Autodesk Fusion 360 part; units mm, degrees
(part 8 of 9)
  spline S40 degree 5 poles (-3.0485, 6.2691) (-3.0485, 6.2692) (-3.0485, 6.2692) (-3.0486, 6.2693) (-3.0487, 6.2695) (-3.0488, 6.2697) (-3.0489, 6.27) (-3.0491, 6.2703) (-3.0493, 6.2707) (-3.0495, 6.271) (-3.0497, 6.2715) (-3.0499, 6.2719) (-3.0502, 6.2724) (-3.0504, 6.2729) (-3.0507, 6.2734) (-3.051, 6.274) (-3.0514, 6.2746) (-3.0517, 6.2752) (-3.0521, 6.2759) (-3.0525, 6.2766) (-3.0529, 6.2773) (-3.0533, 6.2781) (-3.0537, 6.2789) (-3.0542, 6.2797) (-3.0547, 6.2806) (-3.0552, 6.2815) (-3.0557, 6.2824) (-3.0562, 6.2833) (-3.0568, 6.2843) (-3.0574, 6.2853) (-3.058, 6.2863) (-3.0586, 6.2874) (-3.0592, 6.2885) (-3.0599, 6.2896) (-3.0606, 6.2907) (-3.0613, 6.2919) (-3.062, 6.2931) (-3.0627, 6.2943) (-3.0635, 6.2955) (-3.0643, 6.2968) (-3.0651, 6.2981) (-3.0659, 6.2994) (-3.0667, 6.3008) (-3.0676, 6.3022) (-3.0684, 6.3036) (-3.0693, 6.305) (-3.0703, 6.3065) (-3.0712, 6.308) (-3.0722, 6.3095) (-3.0731, 6.311) (-3.0742, 6.3125) (-3.0752, 6.3141) (-3.0762, 6.3157) (-3.0773, 6.3174) (-3.0784, 6.319) (-3.0795, 6.3207) (-3.0806, 6.3224) (-3.0817, 6.3241) (-3.0829, 6.3259) (-3.0841, 6.3276) (-3.0853, 6.3294) (-3.0865, 6.3312) (-3.0878, 6.3331) (-3.0891, 6.3349) (-3.0904, 6.3368) (-3.0917, 6.3387) (-3.093, 6.3406) (-3.0944, 6.3426) (-3.0957, 6.3445) (-3.0971, 6.3465) (-3.0986, 6.3485) (-3.1, 6.3505) (-3.1015, 6.3526) (-3.1029, 6.3546) (-3.1044, 6.3567) (-3.106, 6.3588) (-3.1075, 6.361) (-3.1091, 6.3631) (-3.1107, 6.3653) (-3.1123, 6.3675) (-3.1139, 6.3697) (-3.1156, 6.3719) (-3.1173, 6.3741) (-3.119, 6.3764) (-3.1207, 6.3787) (-3.1224, 6.381) (-3.1242, 6.3833) (-3.126, 6.3856) (-3.1278, 6.388) (-3.1296, 6.3904) (-3.1314, 6.3927) (-3.1333, 6.3951) (-3.1352, 6.3976) (-3.1371, 6.4) (-3.139, 6.4025) (-3.141, 6.4049) (-3.143, 6.4074) (-3.145, 6.4099) (-3.147, 6.4125) (-3.149, 6.415) (-3.1511, 6.4176) (-3.1532, 6.4201) (-3.1553, 6.4227) (-3.1574, 6.4253) (-3.1596, 6.4279) (-3.1617, 6.4306) (-3.1639, 6.4332) (-3.1662, 6.4359) (-3.1684, 6.4386) (-3.1707, 6.4413) (-3.1729, 6.444) (-3.1752, 6.4467) (-3.1776, 6.4494) (-3.1799, 6.4522) (-3.1823, 6.4549) (-3.1847, 6.4577) (-3.1871, 6.4605) (-3.1895, 6.4633) (-3.192, 6.4661) (-3.1945, 6.469) (-3.197, 6.4718) (-3.1995, 6.4747) (-3.202, 6.4776) (-3.2046, 6.4805) (-3.2072, 6.4834) (-3.2098, 6.4863) (-3.2124, 6.4892) (-3.2151, 6.4921) (-3.2178, 6.4951) (-3.2205, 6.498) (-3.2232, 6.501) (-3.2259, 6.504) (-3.2287, 6.507) (-3.2315, 6.51) (-3.2343, 6.513) (-3.2371, 6.5161) (-3.24, 6.5191) (-3.2428, 6.5222) (-3.2457, 6.5252) (-3.2487, 6.5283) (-3.2516, 6.5314) (-3.2546, 6.5345) (-3.2576, 6.5376) (-3.2606, 6.5408) (-3.2636, 6.5439) (-3.2666, 6.547) (-3.2697, 6.5502) (-3.2728, 6.5533) (-3.2759, 6.5565) (-3.2791, 6.5597) (-3.2822, 6.5629) (-3.2854, 6.5661) (-3.2886, 6.5693) (-3.2918, 6.5725) (-3.2951, 6.5758) (-3.2984, 6.579) (-3.3017, 6.5822) (-3.305, 6.5855) (-3.3083, 6.5888) (-3.3117, 6.592) (-3.3151, 6.5953) (-3.3185, 6.5986) (-3.3219, 6.6019) (-3.3253, 6.6052) (-3.3288, 6.6085) (-3.3323, 6.6119) (-3.3358, 6.6152) (-3.3393, 6.6186) (-3.3429, 6.6219) (-3.3465, 6.6253) (-3.3501, 6.6286) (-3.3537, 6.632) (-3.3573, 6.6354) (-3.361, 6.6388) (-3.3647, 6.6422) (-3.3684, 6.6456) (-3.3721, 6.649) (-3.3759, 6.6524) (-3.3797, 6.6558) (-3.3835, 6.6592) (-3.3873, 6.6627) (-3.3911, 6.6661) (-3.395, 6.6695) (-3.3989, 6.673) (-3.4028, 6.6765) (-3.4067, 6.6799) (-3.4107, 6.6834) (-3.4147, 6.6869) (-3.4187, 6.6904) (-3.4227, 6.6939) (-3.4267, 6.6973) (-3.4308, 6.7008) (-3.4349, 6.7044) (-3.439, 6.7079) (-3.4431, 6.7114) (-3.4472, 6.7149) (-3.4514, 6.7184) (-3.4556, 6.722) (-3.4598, 6.7255) (-3.464, 6.729) (-3.4683, 6.7326) (-3.4726, 6.7361) (-3.4769, 6.7397) (-3.4812, 6.7432) (-3.4856, 6.7468) (-3.4899, 6.7504) (-3.4943, 6.7539) (-3.4987, 6.7575) (-3.5031, 6.7611) (-3.5076, 6.7647) (-3.5121, 6.7683) (-3.5166, 6.7719) (-3.5211, 6.7754) (-3.5256, 6.779) (-3.5302, 6.7826) (-3.5348, 6.7862) (-3.5394, 6.7899) (-3.544, 6.7935) (-3.5486, 6.7971) (-3.5533, 6.8007) (-3.558, 6.8043) (-3.5627, 6.8079) (-3.5674, 6.8116) (-3.5722, 6.8152) (-3.577, 6.8188) (-3.5818, 6.8224) (-3.5866, 6.8261) (-3.5914, 6.8297) (-3.5963, 6.8334) (-3.6012, 6.837) (-3.6061, 6.8406) (-3.611, 6.8443) (-3.616, 6.8479) (-3.6209, 6.8516) (-3.6259, 6.8552) (-3.6309, 6.8589) (-3.636, 6.8625) (-3.641, 6.8662) (-3.6461, 6.8698) (-3.6512, 6.8735) (-3.6563, 6.8772) (-3.6604, 6.8801) (-3.6635, 6.8823) (-3.6656, 6.8837) (-3.6666, 6.8845) knots 0 0 0 0 0 0 0.00416667 0.00833333 0.0125 0.01666667 0.02083333 0.025 0.02916667 0.03333333 0.0375 0.04166667 0.04583333 0.05 0.05416667 0.05833333 0.0625 0.06666667 0.07083333 0.075 0.07916667 0.08333333 0.0875 0.09166667 0.09583333 0.1 0.10416667 0.10833333 0.1125 0.11666667 0.12083333 0.125 0.12916667 0.13333333 0.1375 0.14166667 0.14583333 0.15 0.15416667 0.15833333 0.1625 0.16666667 0.17083333 0.175 0.17916667 0.18333333 0.1875 0.19166667 0.19583333 0.2 0.20416667 0.20833333 0.2125 0.21666667 0.22083333 0.225 0.22916667 0.23333333 0.2375 0.24166667 0.24583333 0.25 0.25416667 0.25833333 0.2625 0.26666667 0.27083333 0.275 0.27916667 0.28333333 0.2875 0.29166667 0.29583333 0.3 0.30416667 0.30833333 0.3125 0.31666667 0.32083333 0.325 0.32916667 0.33333333 0.3375 0.34166667 0.34583333 0.35 0.35416667 0.35833333 0.3625 0.36666667 0.37083333 0.375 0.37916667 0.38333333 0.3875 0.39166667 0.39583333 0.4 0.40416667 0.40833333 0.4125 0.41666667 0.42083333 0.425 0.42916667 0.43333333 0.4375 0.44166667 0.44583333 0.45 0.45416667 0.45833333 0.4625 0.46666667 0.47083333 0.475 0.47916667 0.48333333 0.4875 0.49166667 0.49583333 0.5 0.50416667 0.50833333 0.5125 0.51666667 0.52083333 0.525 0.52916667 0.53333333 0.5375 0.54166667 0.54583333 0.55 0.55416667 0.55833333 0.5625 0.56666667 0.57083333 0.575 0.57916667 0.58333333 0.5875 0.59166667 0.59583333 0.6 0.60416667 0.60833333 0.6125 0.61666667 0.62083333 0.625 0.62916667 0.63333333 0.6375 0.64166667 0.64583333 0.65 0.65416667 0.65833333 0.6625 0.66666667 0.67083333 0.675 0.67916667 0.68333333 0.6875 0.69166667 0.69583333 0.7 0.70416667 0.70833333 0.7125 0.71666667 0.72083333 0.725 0.72916667 0.73333333 0.7375 0.74166667 0.74583333 0.75 0.75416667 0.75833333 0.7625 0.76666667 0.77083333 0.775 0.77916667 0.78333333 0.7875 0.79166667 0.79583333 0.8 0.80416667 0.80833333 0.8125 0.81666667 0.82083333 0.825 0.82916667 0.83333333 0.8375 0.84166667 0.84583333 0.85 0.85416667 0.85833333 0.8625 0.86666667 0.87083333 0.875 0.87916667 0.88333333 0.8875 0.89166667 0.89583333 0.9 0.90416667 0.90833333 0.9125 0.91666667 0.92083333 0.925 0.92916667 0.93333333 0.9375 0.94166667 0.94583333 0.95 0.95416667 0.95833333 0.9625 0.96666667 0.97083333 0.975 0.97916667 0.98333333 0.9875 0.99166667 0.99583333 1 1 1 1 1 1
  arc A41 (-3.6666, 6.8845) -> (-4.1288, 6.6176) centre (0, 0) ccw
  spline S41 degree 5 poles (-4.1288, 6.6176) (-4.1287, 6.6163) (-4.1285, 6.6138) (-4.1281, 6.61) (-4.1276, 6.605) (-4.127, 6.5988) (-4.1264, 6.5925) (-4.1258, 6.5863) (-4.1251, 6.5801) (-4.1245, 6.5739) (-4.1238, 6.5677) (-4.1232, 6.5616) (-4.1225, 6.5555) (-4.1218, 6.5494) (-4.1211, 6.5433) (-4.1204, 6.5372) (-4.1197, 6.5312) (-4.119, 6.5251) (-4.1183, 6.5191) (-4.1175, 6.5131) (-4.1168, 6.5072) (-4.116, 6.5012) (-4.1153, 6.4953) (-4.1145, 6.4894) (-4.1137, 6.4835) (-4.1129, 6.4776) (-4.1121, 6.4718) (-4.1113, 6.4659) (-4.1105, 6.4601) (-4.1097, 6.4543) (-4.1089, 6.4486) (-4.108, 6.4428) (-4.1072, 6.4371) (-4.1063, 6.4314) (-4.1055, 6.4257) (-4.1046, 6.42) (-4.1037, 6.4144) (-4.1028, 6.4087) (-4.1019, 6.4031) (-4.101, 6.3975) (-4.1001, 6.392) (-4.0992, 6.3864) (-4.0983, 6.3809) (-4.0974, 6.3754) (-4.0964, 6.3699) (-4.0955, 6.3645) (-4.0945, 6.359) (-4.0936, 6.3536) (-4.0926, 6.3482) (-4.0917, 6.3428) (-4.0907, 6.3375) (-4.0897, 6.3322) (-4.0887, 6.3268) (-4.0877, 6.3216) (-4.0867, 6.3163) (-4.0857, 6.311) (-4.0847, 6.3058) (-4.0837, 6.3006) (-4.0827, 6.2954) (-4.0816, 6.2903) (-4.0806, 6.2851) (-4.0795, 6.28) (-4.0785, 6.2749) (-4.0774, 6.2699) (-4.0764, 6.2648) (-4.0753, 6.2598) (-4.0743, 6.2548) (-4.0732, 6.2498) (-4.0721, 6.2448) (-4.071, 6.2399) (-4.0699, 6.235) (-4.0688, 6.2301) (-4.0677, 6.2252) (-4.0666, 6.2204) (-4.0655, 6.2156) (-4.0644, 6.2108) (-4.0633, 6.206) (-4.0622, 6.2012) (-4.061, 6.1965) (-4.0599, 6.1918) (-4.0588, 6.1871) (-4.0576, 6.1824) (-4.0565, 6.1778) (-4.0553, 6.1732) (-4.0542, 6.1686) (-4.053, 6.164) (-4.0519, 6.1595) (-4.0507, 6.1549) (-4.0496, 6.1504) (-4.0484, 6.146) (-4.0472, 6.1415) (-4.0461, 6.1371) (-4.0449, 6.1327) (-4.0437, 6.1283) (-4.0425, 6.1239) (-4.0413, 6.1196) (-4.0401, 6.1153) (-4.039, 6.111) (-4.0378, 6.1067) (-4.0366, 6.1025) (-4.0354, 6.0983) (-4.0342, 6.0941) (-4.033, 6.0899) (-4.0318, 6.0858) (-4.0306, 6.0817) (-4.0294, 6.0776) (-4.0282, 6.0735) (-4.0269, 6.0695) (-4.0257, 6.0655) (-4.0245, 6.0615) (-4.0233, 6.0575) (-4.0221, 6.0536) (-4.0209, 6.0496) (-4.0197, 6.0457) (-4.0185, 6.0419) (-4.0172, 6.038) (-4.016, 6.0342) (-4.0148, 6.0304) (-4.0136, 6.0266) (-4.0124, 6.0229) (-4.0112, 6.0192) (-4.0099, 6.0155) (-4.0087, 6.0118) (-4.0075, 6.0082) (-4.0063, 6.0046) (-4.0051, 6.001) (-4.0039, 5.9974) (-4.0026, 5.9939) (-4.0014, 5.9904) (-4.0002, 5.9869) (-3.999, 5.9834) (-3.9978, 5.98) (-3.9966, 5.9766) (-3.9954, 5.9732) (-3.9942, 5.9698) (-3.993, 5.9665) (-3.9918, 5.9632) (-3.9906, 5.9599) (-3.9894, 5.9567) (-3.9882, 5.9534) (-3.987, 5.9502) (-3.9858, 5.9471) (-3.9846, 5.9439) (-3.9834, 5.9408) (-3.9822, 5.9377) (-3.981, 5.9346) (-3.9799, 5.9316) (-3.9787, 5.9286) (-3.9775, 5.9256) (-3.9763, 5.9226) (-3.9752, 5.9197) (-3.974, 5.9168) (-3.9729, 5.9139) (-3.9717, 5.9111) (-3.9706, 5.9083) (-3.9694, 5.9055) (-3.9683, 5.9027) (-3.9671, 5.9) (-3.966, 5.8973) (-3.9649, 5.8946) (-3.9638, 5.8919) (-3.9626, 5.8893) (-3.9615, 5.8867) (-3.9604, 5.8841) (-3.9593, 5.8816) (-3.9582, 5.8791) (-3.9572, 5.8766) (-3.9561, 5.8741) (-3.955, 5.8717) (-3.9539, 5.8693) (-3.9529, 5.8669) (-3.9518, 5.8646) (-3.9508, 5.8622) (-3.9497, 5.8599) (-3.9487, 5.8577) (-3.9477, 5.8555) (-3.9466, 5.8532) (-3.9456, 5.8511) (-3.9446, 5.8489) (-3.9436, 5.8468) (-3.9426, 5.8447) (-3.9417, 5.8427) (-3.9407, 5.8406) (-3.9397, 5.8386) (-3.9388, 5.8367) (-3.9378, 5.8347) (-3.9369, 5.8328) (-3.936, 5.8309) (-3.935, 5.8291) (-3.9341, 5.8272) (-3.9332, 5.8254) (-3.9324, 5.8237) (-3.9315, 5.8219) (-3.9306, 5.8202) (-3.9298, 5.8186) (-3.9289, 5.8169) (-3.9281, 5.8153) (-3.9272, 5.8137) (-3.9264, 5.8122) (-3.9256, 5.8106) (-3.9248, 5.8091) (-3.9241, 5.8077) (-3.9233, 5.8062) (-3.9225, 5.8048) (-3.9218, 5.8035) (-3.9211, 5.8021) (-3.9204, 5.8008) (-3.9197, 5.7995) (-3.919, 5.7983) (-3.9183, 5.7971) (-3.9176, 5.7959) (-3.917, 5.7947) (-3.9163, 5.7936) (-3.9157, 5.7925) (-3.9151, 5.7914) (-3.9145, 5.7904) (-3.914, 5.7894) (-3.9134, 5.7884) (-3.9128, 5.7875) (-3.9123, 5.7866) (-3.9118, 5.7857) (-3.9113, 5.7849) (-3.9108, 5.7841) (-3.9104, 5.7833) (-3.9099, 5.7825) (-3.9095, 5.7818) (-3.9091, 5.7811) (-3.9087, 5.7805) (-3.9083, 5.7799) (-3.9079, 5.7793) (-3.9076, 5.7787) (-3.9073, 5.7782) (-3.9069, 5.7777) (-3.9067, 5.7773) (-3.9064, 5.7768) (-3.9061, 5.7764) (-3.9059, 5.7761) (-3.9057, 5.7758) (-3.9055, 5.7755) (-3.9053, 5.7752) (-3.9052, 5.775) (-3.9051, 5.7748) (-3.905, 5.7747) (-3.905, 5.7747) (-3.905, 5.7746) knots -1 -1 -1 -1 -1 -1 -0.99583333 -0.99166667 -0.9875 -0.98333333 -0.97916667 -0.975 -0.97083333 -0.96666667 -0.9625 -0.95833333 -0.95416667 -0.95 -0.94583333 -0.94166667 -0.9375 -0.93333333 -0.92916667 -0.925 -0.92083333 -0.91666667 -0.9125 -0.90833333 -0.90416667 -0.9 -0.89583333 -0.89166667 -0.8875 -0.88333333 -0.87916667 -0.875 -0.87083333 -0.86666667 -0.8625 -0.85833333 -0.85416667 -0.85 -0.84583333 -0.84166667 -0.8375 -0.83333333 -0.82916667 -0.825 -0.82083333 -0.81666667 -0.8125 -0.80833333 -0.80416667 -0.8 -0.79583333 -0.79166667 -0.7875 -0.78333333 -0.77916667 -0.775 -0.77083333 -0.76666667 -0.7625 -0.75833333 -0.75416667 -0.75 -0.74583333 -0.74166667 -0.7375 -0.73333333 -0.72916667 -0.725 -0.72083333 -0.71666667 -0.7125 -0.70833333 -0.70416667 -0.7 -0.69583333 -0.69166667 -0.6875 -0.68333333 -0.67916667 -0.675 -0.67083333 -0.66666667 -0.6625 -0.65833333 -0.65416667 -0.65 -0.64583333 -0.64166667 -0.6375 -0.63333333 -0.62916667 -0.625 -0.62083333 -0.61666667 -0.6125 -0.60833333 -0.60416667 -0.6 -0.59583333 -0.59166667 -0.5875 -0.58333333 -0.57916667 -0.575 -0.57083333 -0.56666667 -0.5625 -0.55833333 -0.55416667 -0.55 -0.54583333 -0.54166667 -0.5375 -0.53333333 -0.52916667 -0.525 -0.52083333 -0.51666667 -0.5125 -0.50833333 -0.50416667 -0.5 -0.49583333 -0.49166667 -0.4875 -0.48333333 -0.47916667 -0.475 -0.47083333 -0.46666667 -0.4625 -0.45833333 -0.45416667 -0.45 -0.44583333 -0.44166667 -0.4375 -0.43333333 -0.42916667 -0.425 -0.42083333 -0.41666667 -0.4125 -0.40833333 -0.40416667 -0.4 -0.39583333 -0.39166667 -0.3875 -0.38333333 -0.37916667 -0.375 -0.37083333 -0.36666667 -0.3625 -0.35833333 -0.35416667 -0.35 -0.34583333 -0.34166667 -0.3375 -0.33333333 -0.32916667 -0.325 -0.32083333 -0.31666667 -0.3125 -0.30833333 -0.30416667 -0.3 -0.29583333 -0.29166667 -0.2875 -0.28333333 -0.27916667 -0.275 -0.27083333 -0.26666667 -0.2625 -0.25833333 -0.25416667 -0.25 -0.24583333 -0.24166667 -0.2375 -0.23333333 -0.22916667 -0.225 -0.22083333 -0.21666667 -0.2125 -0.20833333 -0.20416667 -0.2 -0.19583333 -0.19166667 -0.1875 -0.18333333 -0.17916667 -0.175 -0.17083333 -0.16666667 -0.1625 -0.15833333 -0.15416667 -0.15 -0.14583333 -0.14166667 -0.1375 -0.13333333 -0.12916667 -0.125 -0.12083333 -0.11666667 -0.1125 -0.10833333 -0.10416667 -0.1 -0.09583333 -0.09166667 -0.0875 -0.08333333 -0.07916667 -0.075 -0.07083333 -0.06666667 -0.0625 -0.05833333 -0.05416667 -0.05 -0.04583333 -0.04166667 -0.0375 -0.03333333 -0.02916667 -0.025 -0.02083333 -0.01666667 -0.0125 -0.00833333 -0.00416667 0 0 0 0 0 0
  line L82 (-3.905, 5.7746) -> (-3.9048, 5.7743)
  line L83 (-3.9048, 5.7743) -> (-3.6131, 5.343)
  arc A42 (-3.6131, 5.343) -> (-4.2258, 4.8729) centre (0, 0) ccw
  line L84 (-4.2258, 4.8729) -> (-4.5669, 5.2662)
  line L85 (-4.5669, 5.2662) -> (-4.5672, 5.2665)
  spline S42 degree 5 poles (-4.5672, 5.2665) (-4.5672, 5.2665) (-4.5673, 5.2666) (-4.5673, 5.2667) (-4.5675, 5.2668) (-4.5676, 5.267) (-4.5678, 5.2672) (-4.5681, 5.2675) (-4.5683, 5.2678) (-4.5686, 5.2681) (-4.5689, 5.2684) (-4.5693, 5.2688) (-4.5696, 5.2692) (-4.57, 5.2696) (-4.5705, 5.2701) (-4.5709, 5.2705) (-4.5714, 5.2711) (-4.5719, 5.2716) (-4.5724, 5.2721) (-4.573, 5.2727) (-4.5735, 5.2733) (-4.5741, 5.2739) (-4.5748, 5.2746) (-4.5754, 5.2753) (-4.5761, 5.276) (-4.5768, 5.2767) (-4.5776, 5.2774) (-4.5783, 5.2782) (-4.5791, 5.279) (-4.5799, 5.2798) (-4.5808, 5.2806) (-4.5817, 5.2815) (-4.5826, 5.2824) (-4.5835, 5.2833) (-4.5844, 5.2842) (-4.5854, 5.2852) (-4.5864, 5.2861) (-4.5874, 5.2871) (-4.5885, 5.2881) (-4.5896, 5.2892) (-4.5907, 5.2902) (-4.5918, 5.2913) (-4.593, 5.2924) (-4.5942, 5.2935) (-4.5954, 5.2946) (-4.5966, 5.2958) (-4.5979, 5.2969) (-4.5992, 5.2981) (-4.6005, 5.2993) (-4.6018, 5.3006) (-4.6032, 5.3018) (-4.6046, 5.3031) (-4.606, 5.3043) (-4.6075, 5.3056) (-4.609, 5.307) (-4.6105, 5.3083) (-4.612, 5.3096) (-4.6135, 5.311) (-4.6151, 5.3124) (-4.6167, 5.3138) (-4.6184, 5.3152) (-4.62, 5.3166) (-4.6217, 5.3181) (-4.6234, 5.3195) (-4.6251, 5.321) (-4.6269, 5.3225) (-4.6287, 5.324) (-4.6305, 5.3256) (-4.6323, 5.3271) (-4.6342, 5.3287) (-4.6361, 5.3302) (-4.638, 5.3318) (-4.64, 5.3334) (-4.6419, 5.335) (-4.6439, 5.3366) (-4.6459, 5.3383) (-4.648, 5.3399) (-4.65, 5.3416) (-4.6521, 5.3433) (-4.6543, 5.345) (-4.6564, 5.3467) (-4.6586, 5.3484) (-4.6608, 5.3501) (-4.663, 5.3519) (-4.6653, 5.3536) (-4.6675, 5.3554) (-4.6698, 5.3572) (-4.6722, 5.359) (-4.6745, 5.3608) (-4.6769, 5.3626) (-4.6793, 5.3644) (-4.6817, 5.3663) (-4.6842, 5.3681) (-4.6867, 5.37) (-4.6892, 5.3719) (-4.6917, 5.3737) (-4.6942, 5.3756) (-4.6968, 5.3775) (-4.6994, 5.3795) (-4.7021, 5.3814) (-4.7047, 5.3833) (-4.7074, 5.3853) (-4.7101, 5.3872) (-4.7128, 5.3892) (-4.7156, 5.3911) (-4.7184, 5.3931) (-4.7212, 5.3951) (-4.724, 5.3971) (-4.7269, 5.3991) (-4.7297, 5.4011) (-4.7326, 5.4032) (-4.7356, 5.4052) (-4.7385, 5.4072) (-4.7415, 5.4093) (-4.7445, 5.4114) (-4.7475, 5.4134) (-4.7506, 5.4155) (-4.7537, 5.4176) (-4.7568, 5.4197) (-4.7599, 5.4218) (-4.7631, 5.4239) (-4.7662, 5.426) (-4.7694, 5.4281) (-4.7727, 5.4302) (-4.7759, 5.4324) (-4.7792, 5.4345) (-4.7825, 5.4366) (-4.7858, 5.4388) (-4.7892, 5.4409) (-4.7925, 5.4431) (-4.7959, 5.4453) (-4.7994, 5.4475) (-4.8028, 5.4496) (-4.8063, 5.4518) (-4.8098, 5.454) (-4.8133, 5.4562) (-4.8168, 5.4584) (-4.8204, 5.4606) (-4.824, 5.4628) (-4.8276, 5.4651) (-4.8313, 5.4673) (-4.8349, 5.4695) (-4.8386, 5.4717) (-4.8423, 5.474) (-4.8461, 5.4762) (-4.8498, 5.4785) (-4.8536, 5.4807) (-4.8574, 5.483) (-4.8613, 5.4852) (-4.8651, 5.4875) (-4.869, 5.4898) (-4.8729, 5.492) (-4.8768, 5.4943) (-4.8808, 5.4966) (-4.8847, 5.4989) (-4.8887, 5.5011) (-4.8928, 5.5034) (-4.8968, 5.5057) (-4.9009, 5.508) (-4.905, 5.5103) (-4.9091, 5.5126) (-4.9132, 5.5149) (-4.9174, 5.5172) (-4.9216, 5.5195) (-4.9258, 5.5218) (-4.93, 5.5241) (-4.9343, 5.5264) (-4.9386, 5.5287) (-4.9429, 5.5311) (-4.9472, 5.5334) (-4.9515, 5.5357) (-4.9559, 5.538) (-4.9603, 5.5403) (-4.9647, 5.5427) (-4.9692, 5.545) (-4.9736, 5.5473) (-4.9781, 5.5496) (-4.9826, 5.552) (-4.9872, 5.5543) (-4.9917, 5.5566) (-4.9963, 5.5589) (-5.0009, 5.5613) (-5.0055, 5.5636) (-5.0102, 5.5659) (-5.0148, 5.5683) (-5.0195, 5.5706) (-5.0243, 5.5729) (-5.029, 5.5752) (-5.0338, 5.5776) (-5.0385, 5.5799) (-5.0433, 5.5822) (-5.0482, 5.5846) (-5.053, 5.5869) (-5.0579, 5.5892) (-5.0628, 5.5916) (-5.0677, 5.5939) (-5.0727, 5.5962) (-5.0776, 5.5985) (-5.0826, 5.6009) (-5.0876, 5.6032) (-5.0926, 5.6055) (-5.0977, 5.6078) (-5.1028, 5.6101) (-5.1079, 5.6125) (-5.113, 5.6148) (-5.1181, 5.6171) (-5.1233, 5.6194) (-5.1285, 5.6217) (-5.1337, 5.624) (-5.1389, 5.6263) (-5.1442, 5.6287) (-5.1494, 5.631) (-5.1547, 5.6333) (-5.16, 5.6356) (-5.1654, 5.6379) (-5.1707, 5.6401) (-5.1761, 5.6424) (-5.1815, 5.6447) (-5.1869, 5.647) (-5.1924, 5.6493) (-5.1979, 5.6516) (-5.2033, 5.6539) (-5.2089, 5.6561) (-5.2144, 5.6584) (-5.2199, 5.6607) (-5.2255, 5.6629) (-5.2311, 5.6652) (-5.2367, 5.6675) (-5.2424, 5.6697) (-5.248, 5.672) (-5.2537, 5.6742) (-5.2594, 5.6765) (-5.2651, 5.6787) (-5.2709, 5.681) (-5.2766, 5.6832) (-5.2824, 5.6854) (-5.2882, 5.6876) (-5.294, 5.6899) (-5.2999, 5.6921) (-5.3058, 5.6943) (-5.3117, 5.6965) (-5.3164, 5.6983) (-5.3199, 5.6996) (-5.3223, 5.7005) (-5.3235, 5.7009) knots 0 0 0 0 0 0 0.00416667 0.00833333 0.0125 0.01666667 0.02083333 0.025 0.02916667 0.03333333 0.0375 0.04166667 0.04583333 0.05 0.05416667 0.05833333 0.0625 0.06666667 0.07083333 0.075 0.07916667 0.08333333 0.0875 0.09166667 0.09583333 0.1 0.10416667 0.10833333 0.1125 0.11666667 0.12083333 0.125 0.12916667 0.13333333 0.1375 0.14166667 0.14583333 0.15 0.15416667 0.15833333 0.1625 0.16666667 0.17083333 0.175 0.17916667 0.18333333 0.1875 0.19166667 0.19583333 0.2 0.20416667 0.20833333 0.2125 0.21666667 0.22083333 0.225 0.22916667 0.23333333 0.2375 0.24166667 0.24583333 0.25 0.25416667 0.25833333 0.2625 0.26666667 0.27083333 0.275 0.27916667 0.28333333 0.2875 0.29166667 0.29583333 0.3 0.30416667 0.30833333 0.3125 0.31666667 0.32083333 0.325 0.32916667 0.33333333 0.3375 0.34166667 0.34583333 0.35 0.35416667 0.35833333 0.3625 0.36666667 0.37083333 0.375 0.37916667 0.38333333 0.3875 0.39166667 0.39583333 0.4 0.40416667 0.40833333 0.4125 0.41666667 0.42083333 0.425 0.42916667 0.43333333 0.4375 0.44166667 0.44583333 0.45 0.45416667 0.45833333 0.4625 0.46666667 0.47083333 0.475 0.47916667 0.48333333 0.4875 0.49166667 0.49583333 0.5 0.50416667 0.50833333 0.5125 0.51666667 0.52083333 0.525 0.52916667 0.53333333 0.5375 0.54166667 0.54583333 0.55 0.55416667 0.55833333 0.5625 0.56666667 0.57083333 0.575 0.57916667 0.58333333 0.5875 0.59166667 0.59583333 0.6 0.60416667 0.60833333 0.6125 0.61666667 0.62083333 0.625 0.62916667 0.63333333 0.6375 0.64166667 0.64583333 0.65 0.65416667 0.65833333 0.6625 0.66666667 0.67083333 0.675 0.67916667 0.68333333 0.6875 0.69166667 0.69583333 0.7 0.70416667 0.70833333 0.7125 0.71666667 0.72083333 0.725 0.72916667 0.73333333 0.7375 0.74166667 0.74583333 0.75 0.75416667 0.75833333 0.7625 0.76666667 0.77083333 0.775 0.77916667 0.78333333 0.7875 0.79166667 0.79583333 0.8 0.80416667 0.80833333 0.8125 0.81666667 0.82083333 0.825 0.82916667 0.83333333 0.8375 0.84166667 0.84583333 0.85 0.85416667 0.85833333 0.8625 0.86666667 0.87083333 0.875 0.87916667 0.88333333 0.8875 0.89166667 0.89583333 0.9 0.90416667 0.90833333 0.9125 0.91666667 0.92083333 0.925 0.92916667 0.93333333 0.9375 0.94166667 0.94583333 0.95 0.95416667 0.95833333 0.9625 0.96666667 0.97083333 0.975 0.97916667 0.98333333 0.9875 0.99166667 0.99583333 1 1 1 1 1 1
  arc A43 (-5.3235, 5.7009) -> (-5.7009, 5.3235) centre (0, 0) ccw
  spline S43 degree 5 poles (-5.7009, 5.3235) (-5.7005, 5.3223) (-5.6996, 5.3199) (-5.6983, 5.3164) (-5.6965, 5.3117) (-5.6943, 5.3058) (-5.6921, 5.2999) (-5.6899, 5.294) (-5.6876, 5.2882) (-5.6854, 5.2824) (-5.6832, 5.2766) (-5.681, 5.2709) (-5.6787, 5.2651) (-5.6765, 5.2594) (-5.6742, 5.2537) (-5.672, 5.248) (-5.6697, 5.2424) (-5.6675, 5.2367) (-5.6652, 5.2311) (-5.6629, 5.2255) (-5.6607, 5.2199) (-5.6584, 5.2144) (-5.6561, 5.2089) (-5.6539, 5.2033) (-5.6516, 5.1979) (-5.6493, 5.1924) (-5.647, 5.1869) (-5.6447, 5.1815) (-5.6424, 5.1761) (-5.6401, 5.1707) (-5.6379, 5.1654) (-5.6356, 5.16) (-5.6333, 5.1547) (-5.631, 5.1494) (-5.6287, 5.1442) (-5.6263, 5.1389) (-5.624, 5.1337) (-5.6217, 5.1285) (-5.6194, 5.1233) (-5.6171, 5.1181) (-5.6148, 5.113) (-5.6125, 5.1079) (-5.6101, 5.1028) (-5.6078, 5.0977) (-5.6055, 5.0926) (-5.6032, 5.0876) (-5.6009, 5.0826) (-5.5985, 5.0776) (-5.5962, 5.0727) (-5.5939, 5.0677) (-5.5916, 5.0628) (-5.5892, 5.0579) (-5.5869, 5.053) (-5.5846, 5.0482) (-5.5822, 5.0433) (-5.5799, 5.0385) (-5.5776, 5.0338) (-5.5752, 5.029) (-5.5729, 5.0243) (-5.5706, 5.0195) (-5.5683, 5.0148) (-5.5659, 5.0102) (-5.5636, 5.0055) (-5.5613, 5.0009) (-5.5589, 4.9963) (-5.5566, 4.9917) (-5.5543, 4.9872) (-5.552, 4.9826) (-5.5496, 4.9781) (-5.5473, 4.9736) (-5.545, 4.9692) (-5.5427, 4.9647) (-5.5403, 4.9603) (-5.538, 4.9559) (-5.5357, 4.9515) (-5.5334, 4.9472) (-5.5311, 4.9429) (-5.5287, 4.9386) (-5.5264, 4.9343) (-5.5241, 4.93) (-5.5218, 4.9258) (-5.5195, 4.9216) (-5.5172, 4.9174) (-5.5149, 4.9132) (-5.5126, 4.9091) (-5.5103, 4.905) (-5.508, 4.9009) (-5.5057, 4.8968) (-5.5034, 4.8928) (-5.5011, 4.8887) (-5.4989, 4.8847) (-5.4966, 4.8808) (-5.4943, 4.8768) (-5.492, 4.8729) (-5.4898, 4.869) (-5.4875, 4.8651) (-5.4852, 4.8613) (-5.483, 4.8574) (-5.4807, 4.8536) (-5.4785, 4.8498) (-5.4762, 4.8461) (-5.474, 4.8423) (-5.4717, 4.8386) (-5.4695, 4.8349) (-5.4673, 4.8313) (-5.4651, 4.8276) (-5.4628, 4.824) (-5.4606, 4.8204) (-5.4584, 4.8168) (-5.4562, 4.8133) (-5.454, 4.8098) (-5.4518, 4.8063) (-5.4496, 4.8028) (-5.4475, 4.7994) (-5.4453, 4.7959) (-5.4431, 4.7925) (-5.4409, 4.7892) (-5.4388, 4.7858) (-5.4366, 4.7825) (-5.4345, 4.7792) (-5.4324, 4.7759) (-5.4302, 4.7727) (-5.4281, 4.7694) (-5.426, 4.7662) (-5.4239, 4.7631) (-5.4218, 4.7599) (-5.4197, 4.7568) (-5.4176, 4.7537) (-5.4155, 4.7506) (-5.4134, 4.7475) (-5.4114, 4.7445) (-5.4093, 4.7415) (-5.4072, 4.7385) (-5.4052, 4.7356) (-5.4032, 4.7326) (-5.4011, 4.7297) (-5.3991, 4.7269) (-5.3971, 4.724) (-5.3951, 4.7212) (-5.3931, 4.7184) (-5.3911, 4.7156) (-5.3892, 4.7128) (-5.3872, 4.7101) (-5.3853, 4.7074) (-5.3833, 4.7047) (-5.3814, 4.7021) (-5.3795, 4.6994) (-5.3775, 4.6968) (-5.3756, 4.6942) (-5.3737, 4.6917) (-5.3719, 4.6892) (-5.37, 4.6867) (-5.3681, 4.6842) (-5.3663, 4.6817) (-5.3644, 4.6793) (-5.3626, 4.6769) (-5.3608, 4.6745) (-5.359, 4.6722) (-5.3572, 4.6698) (-5.3554, 4.6675) (-5.3536, 4.6653) (-5.3519, 4.663) (-5.3501, 4.6608) (-5.3484, 4.6586) (-5.3467, 4.6564) (-5.345, 4.6543) (-5.3433, 4.6521) (-5.3416, 4.65) (-5.3399, 4.648) (-5.3383, 4.6459) (-5.3366, 4.6439) (-5.335, 4.6419) (-5.3334, 4.64) (-5.3318, 4.638) (-5.3302, 4.6361) (-5.3287, 4.6342) (-5.3271, 4.6323) (-5.3256, 4.6305) (-5.324, 4.6287) (-5.3225, 4.6269) (-5.321, 4.6251) (-5.3195, 4.6234) (-5.3181, 4.6217) (-5.3166, 4.62) (-5.3152, 4.6184) (-5.3138, 4.6167) (-5.3124, 4.6151) (-5.311, 4.6135) (-5.3096, 4.612) (-5.3083, 4.6105) (-5.307, 4.609) (-5.3056, 4.6075) (-5.3043, 4.606) (-5.3031, 4.6046) (-5.3018, 4.6032) (-5.3006, 4.6018) (-5.2993, 4.6005) (-5.2981, 4.5992) (-5.2969, 4.5979) (-5.2958, 4.5966) (-5.2946, 4.5954) (-5.2935, 4.5942) (-5.2924, 4.593) (-5.2913, 4.5918) (-5.2902, 4.5907) (-5.2892, 4.5896) (-5.2881, 4.5885) (-5.2871, 4.5874) (-5.2861, 4.5864) (-5.2852, 4.5854) (-5.2842, 4.5844) (-5.2833, 4.5835) (-5.2824, 4.5826) (-5.2815, 4.5817) (-5.2806, 4.5808) (-5.2798, 4.5799) (-5.279, 4.5791) (-5.2782, 4.5783) (-5.2774, 4.5776) (-5.2767, 4.5768) (-5.276, 4.5761) (-5.2753, 4.5754) (-5.2746, 4.5748) (-5.2739, 4.5741) (-5.2733, 4.5735) (-5.2727, 4.573) (-5.2721, 4.5724) (-5.2716, 4.5719) (-5.2711, 4.5714) (-5.2705, 4.5709) (-5.2701, 4.5705) (-5.2696, 4.57) (-5.2692, 4.5696) (-5.2688, 4.5693) (-5.2684, 4.5689) (-5.2681, 4.5686) (-5.2678, 4.5683) (-5.2675, 4.5681) (-5.2672, 4.5678) (-5.267, 4.5676) (-5.2668, 4.5675) (-5.2667, 4.5673) (-5.2666, 4.5673) (-5.2665, 4.5672) (-5.2665, 4.5672) knots -1 -1 -1 -1 -1 -1 -0.99583333 -0.99166667 -0.9875 -0.98333333 -0.97916667 -0.975 -0.97083333 -0.96666667 -0.9625 -0.95833333 -0.95416667 -0.95 -0.94583333 -0.94166667 -0.9375 -0.93333333 -0.92916667 -0.925 -0.92083333 -0.91666667 -0.9125 -0.90833333 -0.90416667 -0.9 -0.89583333 -0.89166667 -0.8875 -0.88333333 -0.87916667 -0.875 -0.87083333 -0.86666667 -0.8625 -0.85833333 -0.85416667 -0.85 -0.84583333 -0.84166667 -0.8375 -0.83333333 -0.82916667 -0.825 -0.82083333 -0.81666667 -0.8125 -0.80833333 -0.80416667 -0.8 -0.79583333 -0.79166667 -0.7875 -0.78333333 -0.77916667 -0.775 -0.77083333 -0.76666667 -0.7625 -0.75833333 -0.75416667 -0.75 -0.74583333 -0.74166667 -0.7375 -0.73333333 -0.72916667 -0.725 -0.72083333 -0.71666667 -0.7125 -0.70833333 -0.70416667 -0.7 -0.69583333 -0.69166667 -0.6875 -0.68333333 -0.67916667 -0.675 -0.67083333 -0.66666667 -0.6625 -0.65833333 -0.65416667 -0.65 -0.64583333 -0.64166667 -0.6375 -0.63333333 -0.62916667 -0.625 -0.62083333 -0.61666667 -0.6125 -0.60833333 -0.60416667 -0.6 -0.59583333 -0.59166667 -0.5875 -0.58333333 -0.57916667 -0.575 -0.57083333 -0.56666667 -0.5625 -0.55833333 -0.55416667 -0.55 -0.54583333 -0.54166667 -0.5375 -0.53333333 -0.52916667 -0.525 -0.52083333 -0.51666667 -0.5125 -0.50833333 -0.50416667 -0.5 -0.49583333 -0.49166667 -0.4875 -0.48333333 -0.47916667 -0.475 -0.47083333 -0.46666667 -0.4625 -0.45833333 -0.45416667 -0.45 -0.44583333 -0.44166667 -0.4375 -0.43333333 -0.42916667 -0.425 -0.42083333 -0.41666667 -0.4125 -0.40833333 -0.40416667 -0.4 -0.39583333 -0.39166667 -0.3875 -0.38333333 -0.37916667 -0.375 -0.37083333 -0.36666667 -0.3625 -0.35833333 -0.35416667 -0.35 -0.34583333 -0.34166667 -0.3375 -0.33333333 -0.32916667 -0.325 -0.32083333 -0.31666667 -0.3125 -0.30833333 -0.30416667 -0.3 -0.29583333 -0.29166667 -0.2875 -0.28333333 -0.27916667 -0.275 -0.27083333 -0.26666667 -0.2625 -0.25833333 -0.25416667 -0.25 -0.24583333 -0.24166667 -0.2375 -0.23333333 -0.22916667 -0.225 -0.22083333 -0.21666667 -0.2125 -0.20833333 -0.20416667 -0.2 -0.19583333 -0.19166667 -0.1875 -0.18333333 -0.17916667 -0.175 -0.17083333 -0.16666667 -0.1625 -0.15833333 -0.15416667 -0.15 -0.14583333 -0.14166667 -0.1375 -0.13333333 -0.12916667 -0.125 -0.12083333 -0.11666667 -0.1125 -0.10833333 -0.10416667 -0.1 -0.09583333 -0.09166667 -0.0875 -0.08333333 -0.07916667 -0.075 -0.07083333 -0.06666667 -0.0625 -0.05833333 -0.05416667 -0.05 -0.04583333 -0.04166667 -0.0375 -0.03333333 -0.02916667 -0.025 -0.02083333 -0.01666667 -0.0125 -0.00833333 -0.00416667 0 0 0 0 0 0
  line L86 (-5.2665, 4.5672) -> (-5.2662, 4.5669)
  line L87 (-5.2662, 4.5669) -> (-4.8729, 4.2258)
  arc A44 (-4.8729, 4.2258) -> (-5.343, 3.6131) centre (0, 0) ccw
  line L88 (-5.343, 3.6131) -> (-5.7743, 3.9048)
  line L89 (-5.7743, 3.9048) -> (-5.7746, 3.905)
  spline S44 degree 5 poles (-5.7746, 3.905) (-5.7747, 3.905) (-5.7747, 3.905) (-5.7748, 3.9051) (-5.775, 3.9052) (-5.7752, 3.9053) (-5.7755, 3.9055) (-5.7758, 3.9057) (-5.7761, 3.9059) (-5.7764, 3.9061) (-5.7768, 3.9064) (-5.7773, 3.9067) (-5.7777, 3.9069) (-5.7782, 3.9073) (-5.7787, 3.9076) (-5.7793, 3.9079) (-5.7799, 3.9083) (-5.7805, 3.9087) (-5.7811, 3.9091) (-5.7818, 3.9095) (-5.7825, 3.9099) (-5.7833, 3.9104) (-5.7841, 3.9108) (-5.7849, 3.9113) (-5.7857, 3.9118) (-5.7866, 3.9123) (-5.7875, 3.9128) (-5.7884, 3.9134) (-5.7894, 3.914) (-5.7904, 3.9145) (-5.7914, 3.9151) (-5.7925, 3.9157) (-5.7936, 3.9163) (-5.7947, 3.917) (-5.7959, 3.9176) (-5.7971, 3.9183) (-5.7983, 3.919) (-5.7995, 3.9197) (-5.8008, 3.9204) (-5.8021, 3.9211) (-5.8035, 3.9218) (-5.8048, 3.9225) (-5.8062, 3.9233) (-5.8077, 3.9241) (-5.8091, 3.9248) (-5.8106, 3.9256) (-5.8122, 3.9264) (-5.8137, 3.9272) (-5.8153, 3.9281) (-5.8169, 3.9289) (-5.8186, 3.9298) (-5.8202, 3.9306) (-5.8219, 3.9315) (-5.8237, 3.9324) (-5.8254, 3.9332) (-5.8272, 3.9341) (-5.8291, 3.935) (-5.8309, 3.936) (-5.8328, 3.9369) (-5.8347, 3.9378) (-5.8367, 3.9388) (-5.8386, 3.9397) (-5.8406, 3.9407) (-5.8427, 3.9417) (-5.8447, 3.9426) (-5.8468, 3.9436) (-5.8489, 3.9446) (-5.8511, 3.9456) (-5.8532, 3.9466) (-5.8555, 3.9477) (-5.8577, 3.9487) (-5.8599, 3.9497) (-5.8622, 3.9508) (-5.8646, 3.9518) (-5.8669, 3.9529) (-5.8693, 3.9539) (-5.8717, 3.955) (-5.8741, 3.9561) (-5.8766, 3.9572) (-5.8791, 3.9582) (-5.8816, 3.9593) (-5.8841, 3.9604) (-5.8867, 3.9615) (-5.8893, 3.9626) (-5.8919, 3.9638) (-5.8946, 3.9649) (-5.8973, 3.966) (-5.9, 3.9671) (-5.9027, 3.9683) (-5.9055, 3.9694) (-5.9083, 3.9706) (-5.9111, 3.9717) (-5.9139, 3.9729) (-5.9168, 3.974) (-5.9197, 3.9752) (-5.9226, 3.9763) (-5.9256, 3.9775) (-5.9286, 3.9787) (-5.9316, 3.9799) (-5.9346, 3.981) (-5.9377, 3.9822) (-5.9408, 3.9834) (-5.9439, 3.9846) (-5.9471, 3.9858) (-5.9502, 3.987) (-5.9534, 3.9882) (-5.9567, 3.9894) (-5.9599, 3.9906) (-5.9632, 3.9918) (-5.9665, 3.993) (-5.9698, 3.9942) (-5.9732, 3.9954) (-5.9766, 3.9966) (-5.98, 3.9978) (-5.9834, 3.999) (-5.9869, 4.0002) (-5.9904, 4.0014) (-5.9939, 4.0026) (-5.9974, 4.0039) (-6.001, 4.0051) (-6.0046, 4.0063) (-6.0082, 4.0075) (-6.0118, 4.0087) (-6.0155, 4.0099) (-6.0192, 4.0112) (-6.0229, 4.0124) (-6.0266, 4.0136) (-6.0304, 4.0148) (-6.0342, 4.016) (-6.038, 4.0172) (-6.0419, 4.0185) (-6.0457, 4.0197) (-6.0496, 4.0209) (-6.0536, 4.0221) (-6.0575, 4.0233) (-6.0615, 4.0245) (-6.0655, 4.0257) (-6.0695, 4.0269) (-6.0735, 4.0282) (-6.0776, 4.0294) (-6.0817, 4.0306) (-6.0858, 4.0318) (-6.0899, 4.033) (-6.0941, 4.0342) (-6.0983, 4.0354) (-6.1025, 4.0366) (-6.1067, 4.0378) (-6.111, 4.039) (-6.1153, 4.0401) (-6.1196, 4.0413) (-6.1239, 4.0425) (-6.1283, 4.0437) (-6.1327, 4.0449) (-6.1371, 4.0461) (-6.1415, 4.0472) (-6.146, 4.0484) (-6.1504, 4.0496) (-6.1549, 4.0507) (-6.1595, 4.0519) (-6.164, 4.053) (-6.1686, 4.0542) (-6.1732, 4.0553) (-6.1778, 4.0565) (-6.1824, 4.0576) (-6.1871, 4.0588) (-6.1918, 4.0599) (-6.1965, 4.061) (-6.2012, 4.0622) (-6.206, 4.0633) (-6.2108, 4.0644) (-6.2156, 4.0655) (-6.2204, 4.0666) (-6.2252, 4.0677) (-6.2301, 4.0688) (-6.235, 4.0699) (-6.2399, 4.071) (-6.2448, 4.0721) (-6.2498, 4.0732) (-6.2548, 4.0743) (-6.2598, 4.0753) (-6.2648, 4.0764) (-6.2699, 4.0774) (-6.2749, 4.0785) (-6.28, 4.0795) (-6.2851, 4.0806) (-6.2903, 4.0816) (-6.2954, 4.0827) (-6.3006, 4.0837) (-6.3058, 4.0847) (-6.311, 4.0857) (-6.3163, 4.0867) (-6.3216, 4.0877) (-6.3268, 4.0887) (-6.3322, 4.0897) (-6.3375, 4.0907) (-6.3428, 4.0917) (-6.3482, 4.0926) (-6.3536, 4.0936) (-6.359, 4.0945) (-6.3645, 4.0955) (-6.3699, 4.0964) (-6.3754, 4.0974) (-6.3809, 4.0983) (-6.3864, 4.0992) (-6.392, 4.1001) (-6.3975, 4.101) (-6.4031, 4.1019) (-6.4087, 4.1028) (-6.4144, 4.1037) (-6.42, 4.1046) (-6.4257, 4.1055) (-6.4314, 4.1063) (-6.4371, 4.1072) (-6.4428, 4.108) (-6.4486, 4.1089) (-6.4543, 4.1097) (-6.4601, 4.1105) (-6.4659, 4.1113) (-6.4718, 4.1121) (-6.4776, 4.1129) (-6.4835, 4.1137) (-6.4894, 4.1145) (-6.4953, 4.1153) (-6.5012, 4.116) (-6.5072, 4.1168) (-6.5131, 4.1175) (-6.5191, 4.1183) (-6.5251, 4.119) (-6.5312, 4.1197) (-6.5372, 4.1204) (-6.5433, 4.1211) (-6.5494, 4.1218) (-6.5555, 4.1225) (-6.5616, 4.1232) (-6.5677, 4.1238) (-6.5739, 4.1245) (-6.5801, 4.1251) (-6.5863, 4.1258) (-6.5925, 4.1264) (-6.5988, 4.127) (-6.605, 4.1276) (-6.61, 4.1281) (-6.6138, 4.1285) (-6.6163, 4.1287) (-6.6176, 4.1288) knots 0 0 0 0 0 0 0.00416667 0.00833333 0.0125 0.01666667 0.02083333 0.025 0.02916667 0.03333333 0.0375 0.04166667 0.04583333 0.05 0.05416667 0.05833333 0.0625 0.06666667 0.07083333 0.075 0.07916667 0.08333333 0.0875 0.09166667 0.09583333 0.1 0.10416667 0.10833333 0.1125 0.11666667 0.12083333 0.125 0.12916667 0.13333333 0.1375 0.14166667 0.14583333 0.15 0.15416667 0.15833333 0.1625 0.16666667 0.17083333 0.175 0.17916667 0.18333333 0.1875 0.19166667 0.19583333 0.2 0.20416667 0.20833333 0.2125 0.21666667 0.22083333 0.225 0.22916667 0.23333333 0.2375 0.24166667 0.24583333 0.25 0.25416667 0.25833333 0.2625 0.26666667 0.27083333 0.275 0.27916667 0.28333333 0.2875 0.29166667 0.29583333 0.3 0.30416667 0.30833333 0.3125 0.31666667 0.32083333 0.325 0.32916667 0.33333333 0.3375 0.34166667 0.34583333 0.35 0.35416667 0.35833333 0.3625 0.36666667 0.37083333 0.375 0.37916667 0.38333333 0.3875 0.39166667 0.39583333 0.4 0.40416667 0.40833333 0.4125 0.41666667 0.42083333 0.425 0.42916667 0.43333333 0.4375 0.44166667 0.44583333 0.45 0.45416667 0.45833333 0.4625 0.46666667 0.47083333 0.475 0.47916667 0.48333333 0.4875 0.49166667 0.49583333 0.5 0.50416667 0.50833333 0.5125 0.51666667 0.52083333 0.525 0.52916667 0.53333333 0.5375 0.54166667 0.54583333 0.55 0.55416667 0.55833333 0.5625 0.56666667 0.57083333 0.575 0.57916667 0.58333333 0.5875 0.59166667 0.59583333 0.6 0.60416667 0.60833333 0.6125 0.61666667 0.62083333 0.625 0.62916667 0.63333333 0.6375 0.64166667 0.64583333 0.65 0.65416667 0.65833333 0.6625 0.66666667 0.67083333 0.675 0.67916667 0.68333333 0.6875 0.69166667 0.69583333 0.7 0.70416667 0.70833333 0.7125 0.71666667 0.72083333 0.725 0.72916667 0.73333333 0.7375 0.74166667 0.74583333 0.75 0.75416667 0.75833333 0.7625 0.76666667 0.77083333 0.775 0.77916667 0.78333333 0.7875 0.79166667 0.79583333 0.8 0.80416667 0.80833333 0.8125 0.81666667 0.82083333 0.825 0.82916667 0.83333333 0.8375 0.84166667 0.84583333 0.85 0.85416667 0.85833333 0.8625 0.86666667 0.87083333 0.875 0.87916667 0.88333333 0.8875 0.89166667 0.89583333 0.9 0.90416667 0.90833333 0.9125 0.91666667 0.92083333 0.925 0.92916667 0.93333333 0.9375 0.94166667 0.94583333 0.95 0.95416667 0.95833333 0.9625 0.96666667 0.97083333 0.975 0.97916667 0.98333333 0.9875 0.99166667 0.99583333 1 1 1 1 1 1
  arc A45 (-6.6176, 4.1288) -> (-6.8845, 3.6666) centre (0, 0) ccw
  spline S45 degree 5 poles (-6.8845, 3.6666) (-6.8837, 3.6656) (-6.8823, 3.6635) (-6.8801, 3.6604) (-6.8772, 3.6563) (-6.8735, 3.6512) (-6.8698, 3.6461) (-6.8662, 3.641) (-6.8625, 3.636) (-6.8589, 3.6309) (-6.8552, 3.6259) (-6.8516, 3.6209) (-6.8479, 3.616) (-6.8443, 3.611) (-6.8406, 3.6061) (-6.837, 3.6012) (-6.8334, 3.5963) (-6.8297, 3.5914) (-6.8261, 3.5866) (-6.8224, 3.5818) (-6.8188, 3.577) (-6.8152, 3.5722) (-6.8116, 3.5674) (-6.8079, 3.5627) (-6.8043, 3.558) (-6.8007, 3.5533) (-6.7971, 3.5486) (-6.7935, 3.544) (-6.7899, 3.5394) (-6.7862, 3.5348) (-6.7826, 3.5302) (-6.779, 3.5256) (-6.7754, 3.5211) (-6.7719, 3.5166) (-6.7683, 3.5121) (-6.7647, 3.5076) (-6.7611, 3.5031) (-6.7575, 3.4987) (-6.7539, 3.4943) (-6.7504, 3.4899) (-6.7468, 3.4856) (-6.7432, 3.4812) (-6.7397, 3.4769) (-6.7361, 3.4726) (-6.7326, 3.4683) (-6.729, 3.464) (-6.7255, 3.4598) (-6.722, 3.4556) (-6.7184, 3.4514) (-6.7149, 3.4472) (-6.7114, 3.4431) (-6.7079, 3.439) (-6.7044, 3.4349) (-6.7008, 3.4308) (-6.6973, 3.4267) (-6.6939, 3.4227) (-6.6904, 3.4187) (-6.6869, 3.4147) (-6.6834, 3.4107) (-6.6799, 3.4067) (-6.6765, 3.4028) (-6.673, 3.3989) (-6.6695, 3.395) (-6.6661, 3.3911) (-6.6627, 3.3873) (-6.6592, 3.3835) (-6.6558, 3.3797) (-6.6524, 3.3759) (-6.649, 3.3721) (-6.6456, 3.3684) (-6.6422, 3.3647) (-6.6388, 3.361) (-6.6354, 3.3573) (-6.632, 3.3537) (-6.6286, 3.3501) (-6.6253, 3.3465) (-6.6219, 3.3429) (-6.6186, 3.3393) (-6.6152, 3.3358) (-6.6119, 3.3323) (-6.6085, 3.3288) (-6.6052, 3.3253) (-6.6019, 3.3219) (-6.5986, 3.3185) (-6.5953, 3.3151) (-6.592, 3.3117) (-6.5888, 3.3083) (-6.5855, 3.305) (-6.5822, 3.3017) (-6.579, 3.2984) (-6.5758, 3.2951) (-6.5725, 3.2918) (-6.5693, 3.2886) (-6.5661, 3.2854) (-6.5629, 3.2822) (-6.5597, 3.2791) (-6.5565, 3.2759) (-6.5533, 3.2728) (-6.5502, 3.2697) (-6.547, 3.2666) (-6.5439, 3.2636) (-6.5408, 3.2606) (-6.5376, 3.2576) (-6.5345, 3.2546) (-6.5314, 3.2516) (-6.5283, 3.2487) (-6.5252, 3.2457) (-6.5222, 3.2428) (-6.5191, 3.24) (-6.5161, 3.2371) (-6.513, 3.2343) (-6.51, 3.2315) (-6.507, 3.2287) (-6.504, 3.2259) (-6.501, 3.2232) (-6.498, 3.2205) (-6.4951, 3.2178) (-6.4921, 3.2151) (-6.4892, 3.2124) (-6.4863, 3.2098) (-6.4834, 3.2072) (-6.4805, 3.2046) (-6.4776, 3.202) (-6.4747, 3.1995) (-6.4718, 3.197) (-6.469, 3.1945) (-6.4661, 3.192) (-6.4633, 3.1895) (-6.4605, 3.1871) (-6.4577, 3.1847) (-6.4549, 3.1823) (-6.4522, 3.1799) (-6.4494, 3.1776) (-6.4467, 3.1752) (-6.444, 3.1729) (-6.4413, 3.1707) (-6.4386, 3.1684) (-6.4359, 3.1662) (-6.4332, 3.1639) (-6.4306, 3.1617) (-6.4279, 3.1596) (-6.4253, 3.1574) (-6.4227, 3.1553) (-6.4201, 3.1532) (-6.4176, 3.1511) (-6.415, 3.149) (-6.4125, 3.147) (-6.4099, 3.145) (-6.4074, 3.143) (-6.4049, 3.141) (-6.4025, 3.139) (-6.4, 3.1371) (-6.3976, 3.1352) (-6.3951, 3.1333) (-6.3927, 3.1314) (-6.3904, 3.1296) (-6.388, 3.1278) (-6.3856, 3.126) (-6.3833, 3.1242) (-6.381, 3.1224) (-6.3787, 3.1207) (-6.3764, 3.119) (-6.3741, 3.1173) (-6.3719, 3.1156) (-6.3697, 3.1139) (-6.3675, 3.1123) (-6.3653, 3.1107) (-6.3631, 3.1091) (-6.361, 3.1075) (-6.3588, 3.106) (-6.3567, 3.1044) (-6.3546, 3.1029) (-6.3526, 3.1015) (-6.3505, 3.1) (-6.3485, 3.0986) (-6.3465, 3.0971) (-6.3445, 3.0957) (-6.3426, 3.0944) (-6.3406, 3.093) (-6.3387, 3.0917) (-6.3368, 3.0904) (-6.3349, 3.0891) (-6.3331, 3.0878) (-6.3312, 3.0865) (-6.3294, 3.0853) (-6.3276, 3.0841) (-6.3259, 3.0829) (-6.3241, 3.0817) (-6.3224, 3.0806) (-6.3207, 3.0795) (-6.319, 3.0784) (-6.3174, 3.0773) (-6.3157, 3.0762) (-6.3141, 3.0752) (-6.3125, 3.0742) (-6.311, 3.0731) (-6.3095, 3.0722) (-6.308, 3.0712) (-6.3065, 3.0703) (-6.305, 3.0693) (-6.3036, 3.0684) (-6.3022, 3.0676) (-6.3008, 3.0667) (-6.2994, 3.0659) (-6.2981, 3.0651) (-6.2968, 3.0643) (-6.2955, 3.0635) (-6.2943, 3.0627) (-6.2931, 3.062) (-6.2919, 3.0613) (-6.2907, 3.0606) (-6.2896, 3.0599) (-6.2885, 3.0592) (-6.2874, 3.0586) (-6.2863, 3.058) (-6.2853, 3.0574) (-6.2843, 3.0568) (-6.2833, 3.0562) (-6.2824, 3.0557) (-6.2815, 3.0552) (-6.2806, 3.0547) (-6.2797, 3.0542) (-6.2789, 3.0537) (-6.2781, 3.0533) (-6.2773, 3.0529) (-6.2766, 3.0525) (-6.2759, 3.0521) (-6.2752, 3.0517) (-6.2746, 3.0514) (-6.274, 3.051) (-6.2734, 3.0507) (-6.2729, 3.0504) (-6.2724, 3.0502) (-6.2719, 3.0499) (-6.2715, 3.0497) (-6.271, 3.0495) (-6.2707, 3.0493) (-6.2703, 3.0491) (-6.27, 3.0489) (-6.2697, 3.0488) (-6.2695, 3.0487) (-6.2693, 3.0486) (-6.2692, 3.0485) (-6.2692, 3.0485) (-6.2691, 3.0485) knots -1 -1 -1 -1 -1 -1 -0.99583333 -0.99166667 -0.9875 -0.98333333 -0.97916667 -0.975 -0.97083333 -0.96666667 -0.9625 -0.95833333 -0.95416667 -0.95 -0.94583333 -0.94166667 -0.9375 -0.93333333 -0.92916667 -0.925 -0.92083333 -0.91666667 -0.9125 -0.90833333 -0.90416667 -0.9 -0.89583333 -0.89166667 -0.8875 -0.88333333 -0.87916667 -0.875 -0.87083333 -0.86666667 -0.8625 -0.85833333 -0.85416667 -0.85 -0.84583333 -0.84166667 -0.8375 -0.83333333 -0.82916667 -0.825 -0.82083333 -0.81666667 -0.8125 -0.80833333 -0.80416667 -0.8 -0.79583333 -0.79166667 -0.7875 -0.78333333 -0.77916667 -0.775 -0.77083333 -0.76666667 -0.7625 -0.75833333 -0.75416667 -0.75 -0.74583333 -0.74166667 -0.7375 -0.73333333 -0.72916667 -0.725 -0.72083333 -0.71666667 -0.7125 -0.70833333 -0.70416667 -0.7 -0.69583333 -0.69166667 -0.6875 -0.68333333 -0.67916667 -0.675 -0.67083333 -0.66666667 -0.6625 -0.65833333 -0.65416667 -0.65 -0.64583333 -0.64166667 -0.6375 -0.63333333 -0.62916667 -0.625 -0.62083333 -0.61666667 -0.6125 -0.60833333 -0.60416667 -0.6 -0.59583333 -0.59166667 -0.5875 -0.58333333 -0.57916667 -0.575 -0.57083333 -0.56666667 -0.5625 -0.55833333 -0.55416667 -0.55 -0.54583333 -0.54166667 -0.5375 -0.53333333 -0.52916667 -0.525 -0.52083333 -0.51666667 -0.5125 -0.50833333 -0.50416667 -0.5 -0.49583333 -0.49166667 -0.4875 -0.48333333 -0.47916667 -0.475 -0.47083333 -0.46666667 -0.4625 -0.45833333 -0.45416667 -0.45 -0.44583333 -0.44166667 -0.4375 -0.43333333 -0.42916667 -0.425 -0.42083333 -0.41666667 -0.4125 -0.40833333 -0.40416667 -0.4 -0.39583333 -0.39166667 -0.3875 -0.38333333 -0.37916667 -0.375 -0.37083333 -0.36666667 -0.3625 -0.35833333 -0.35416667 -0.35 -0.34583333 -0.34166667 -0.3375 -0.33333333 -0.32916667 -0.325 -0.32083333 -0.31666667 -0.3125 -0.30833333 -0.30416667 -0.3 -0.29583333 -0.29166667 -0.2875 -0.28333333 -0.27916667 -0.275 -0.27083333 -0.26666667 -0.2625 -0.25833333 -0.25416667 -0.25 -0.24583333 -0.24166667 -0.2375 -0.23333333 -0.22916667 -0.225 -0.22083333 -0.21666667 -0.2125 -0.20833333 -0.20416667 -0.2 -0.19583333 -0.19166667 -0.1875 -0.18333333 -0.17916667 -0.175 -0.17083333 -0.16666667 -0.1625 -0.15833333 -0.15416667 -0.15 -0.14583333 -0.14166667 -0.1375 -0.13333333 -0.12916667 -0.125 -0.12083333 -0.11666667 -0.1125 -0.10833333 -0.10416667 -0.1 -0.09583333 -0.09166667 -0.0875 -0.08333333 -0.07916667 -0.075 -0.07083333 -0.06666667 -0.0625 -0.05833333 -0.05416667 -0.05 -0.04583333 -0.04166667 -0.0375 -0.03333333 -0.02916667 -0.025 -0.02083333 -0.01666667 -0.0125 -0.00833333 -0.00416667 0 0 0 0 0 0
  line L90 (-6.2691, 3.0485) -> (-6.2688, 3.0483)
  line L91 (-6.2688, 3.0483) -> (-5.8006, 2.8206)
  arc A46 (-5.8006, 2.8206) -> (-6.0961, 2.1071) centre (0, 0) ccw
  line L92 (-6.0961, 2.1071) -> (-6.5882, 2.2772)
  line L93 (-6.5882, 2.2772) -> (-6.5886, 2.2773)
  spline S46 degree 5 poles (-6.5886, 2.2773) (-6.5886, 2.2773) (-6.5887, 2.2774) (-6.5888, 2.2774) (-6.5889, 2.2775) (-6.5892, 2.2775) (-6.5895, 2.2776) (-6.5898, 2.2777) (-6.5902, 2.2779) (-6.5906, 2.278) (-6.591, 2.2781) (-6.5915, 2.2783) (-6.592, 2.2784) (-6.5926, 2.2786) (-6.5932, 2.2788) (-6.5938, 2.279) (-6.5945, 2.2792) (-6.5952, 2.2794) (-6.5959, 2.2796) (-6.5967, 2.2798) (-6.5975, 2.28) (-6.5983, 2.2803) (-6.5992, 2.2805) (-6.6001, 2.2808) (-6.601, 2.2811) (-6.602, 2.2813) (-6.603, 2.2816) (-6.6041, 2.2819) (-6.6051, 2.2822) (-6.6063, 2.2825) (-6.6074, 2.2828) (-6.6086, 2.2831) (-6.6098, 2.2834) (-6.6111, 2.2837) (-6.6123, 2.2841) (-6.6137, 2.2844) (-6.615, 2.2847) (-6.6164, 2.2851) (-6.6178, 2.2854) (-6.6193, 2.2858) (-6.6208, 2.2861) (-6.6223, 2.2865) (-6.6238, 2.2868) (-6.6254, 2.2872) (-6.627, 2.2876) (-6.6287, 2.288) (-6.6304, 2.2883) (-6.6321, 2.2887) (-6.6338, 2.2891) (-6.6356, 2.2895) (-6.6374, 2.2899) (-6.6392, 2.2903) (-6.6411, 2.2907) (-6.643, 2.2911) (-6.6449, 2.2915) (-6.6469, 2.2919) (-6.6489, 2.2923) (-6.6509, 2.2927) (-6.653, 2.2931) (-6.6551, 2.2935) (-6.6572, 2.2939) (-6.6594, 2.2943) (-6.6615, 2.2947) (-6.6638, 2.2952) (-6.666, 2.2956) (-6.6683, 2.296) (-6.6706, 2.2964) (-6.6729, 2.2968) (-6.6753, 2.2972) (-6.6777, 2.2976) (-6.6801, 2.2981) (-6.6825, 2.2985) (-6.685, 2.2989) (-6.6875, 2.2993) (-6.6901, 2.2997) (-6.6926, 2.3001) (-6.6952, 2.3005) (-6.6979, 2.3009) (-6.7005, 2.3014) (-6.7032, 2.3018) (-6.7059, 2.3022) (-6.7087, 2.3026) (-6.7114, 2.303) (-6.7142, 2.3034) (-6.7171, 2.3038) (-6.7199, 2.3042) (-6.7228, 2.3045) (-6.7257, 2.3049) (-6.7286, 2.3053) (-6.7316, 2.3057) (-6.7346, 2.3061) (-6.7376, 2.3065) (-6.7407, 2.3068) (-6.7438, 2.3072) (-6.7469, 2.3076) (-6.75, 2.308) (-6.7532, 2.3083) (-6.7563, 2.3087) (-6.7596, 2.309) (-6.7628, 2.3094) (-6.7661, 2.3097) (-6.7694, 2.3101) (-6.7727, 2.3104) (-6.776, 2.3107) (-6.7794, 2.3111) (-6.7828, 2.3114) (-6.7862, 2.3117) (-6.7897, 2.312) (-6.7931, 2.3124) (-6.7966, 2.3127) (-6.8002, 2.313) (-6.8037, 2.3133) (-6.8073, 2.3135) (-6.8109, 2.3138) (-6.8145, 2.3141) (-6.8182, 2.3144) (-6.8219, 2.3147) (-6.8256, 2.3149) (-6.8293, 2.3152) (-6.8331, 2.3154) (-6.8369, 2.3157) (-6.8407, 2.3159) (-6.8445, 2.3161) (-6.8484, 2.3164) (-6.8523, 2.3166) (-6.8562, 2.3168) (-6.8601, 2.317) (-6.864, 2.3172) (-6.868, 2.3174) (-6.872, 2.3176) (-6.8761, 2.3178) (-6.8801, 2.318) (-6.8842, 2.3181) (-6.8883, 2.3183) (-6.8924, 2.3184) (-6.8966, 2.3186) (-6.9007, 2.3187) (-6.9049, 2.3188) (-6.9091, 2.319) (-6.9134, 2.3191) (-6.9176, 2.3192) (-6.9219, 2.3193) (-6.9262, 2.3194) (-6.9306, 2.3194) (-6.9349, 2.3195) (-6.9393, 2.3196) (-6.9437, 2.3196) (-6.9481, 2.3197) (-6.9526, 2.3197) (-6.9571, 2.3198) (-6.9616, 2.3198) (-6.9661, 2.3198) (-6.9706, 2.3198) (-6.9752, 2.3198) (-6.9797, 2.3198) (-6.9843, 2.3198) (-6.989, 2.3197) (-6.9936, 2.3197) (-6.9983, 2.3196) (-7.003, 2.3196) (-7.0077, 2.3195) (-7.0124, 2.3194) (-7.0172, 2.3193) (-7.022, 2.3192) (-7.0268, 2.3191) (-7.0316, 2.319) (-7.0364, 2.3189) (-7.0413, 2.3188) (-7.0462, 2.3186) (-7.0511, 2.3184) (-7.056, 2.3183) (-7.061, 2.3181) (-7.0659, 2.3179) (-7.0709, 2.3177) (-7.0759, 2.3175) (-7.0809, 2.3173) (-7.086, 2.3171) (-7.0911, 2.3168) (-7.0962, 2.3166) (-7.1013, 2.3163) (-7.1064, 2.316) (-7.1115, 2.3157) (-7.1167, 2.3155) (-7.1219, 2.3151) (-7.1271, 2.3148) (-7.1323, 2.3145) (-7.1376, 2.3142) (-7.1429, 2.3138) (-7.1482, 2.3134) (-7.1535, 2.3131) (-7.1588, 2.3127) (-7.1641, 2.3123) (-7.1695, 2.3119) (-7.1749, 2.3115) (-7.1803, 2.311) (-7.1857, 2.3106) (-7.1912, 2.3101) (-7.1966, 2.3097) (-7.2021, 2.3092) (-7.2076, 2.3087) (-7.2131, 2.3082) (-7.2186, 2.3077) (-7.2242, 2.3071) (-7.2298, 2.3066) (-7.2354, 2.3061) (-7.241, 2.3055) (-7.2466, 2.3049) (-7.2523, 2.3043) (-7.2579, 2.3037) (-7.2636, 2.3031) (-7.2693, 2.3025) (-7.275, 2.3018) (-7.2807, 2.3012) (-7.2865, 2.3005) (-7.2923, 2.2998) (-7.2981, 2.2991) (-7.3039, 2.2984) (-7.3097, 2.2977) (-7.3155, 2.297) (-7.3214, 2.2962) (-7.3273, 2.2955) (-7.3332, 2.2947) (-7.3391, 2.2939) (-7.345, 2.2931) (-7.3509, 2.2923) (-7.3569, 2.2915) (-7.3629, 2.2907) (-7.3689, 2.2898) (-7.3749, 2.2889) (-7.3809, 2.2881) (-7.3869, 2.2872) (-7.393, 2.2863) (-7.3991, 2.2854) (-7.4052, 2.2844) (-7.4113, 2.2835) (-7.4174, 2.2825) (-7.4236, 2.2815) (-7.4297, 2.2805) (-7.4359, 2.2795) (-7.4421, 2.2785) (-7.4483, 2.2775) (-7.4533, 2.2767) (-7.457, 2.276) (-7.4595, 2.2756) (-7.4607, 2.2754) knots 0 0 0 0 0 0 0.00416667 0.00833333 0.0125 0.01666667 0.02083333 0.025 0.02916667 0.03333333 0.0375 0.04166667 0.04583333 0.05 0.05416667 0.05833333 0.0625 0.06666667 0.07083333 0.075 0.07916667 0.08333333 0.0875 0.09166667 0.09583333 0.1 0.10416667 0.10833333 0.1125 0.11666667 0.12083333 0.125 0.12916667 0.13333333 0.1375 0.14166667 0.14583333 0.15 0.15416667 0.15833333 0.1625 0.16666667 0.17083333 0.175 0.17916667 0.18333333 0.1875 0.19166667 0.19583333 0.2 0.20416667 0.20833333 0.2125 0.21666667 0.22083333 0.225 0.22916667 0.23333333 0.2375 0.24166667 0.24583333 0.25 0.25416667 0.25833333 0.2625 0.26666667 0.27083333 0.275 0.27916667 0.28333333 0.2875 0.29166667 0.29583333 0.3 0.30416667 0.30833333 0.3125 0.31666667 0.32083333 0.325 0.32916667 0.33333333 0.3375 0.34166667 0.34583333 0.35 0.35416667 0.35833333 0.3625 0.36666667 0.37083333 0.375 0.37916667 0.38333333 0.3875 0.39166667 0.39583333 0.4 0.40416667 0.40833333 0.4125 0.41666667 0.42083333 0.425 0.42916667 0.43333333 0.4375 0.44166667 0.44583333 0.45 0.45416667 0.45833333 0.4625 0.46666667 0.47083333 0.475 0.47916667 0.48333333 0.4875 0.49166667 0.49583333 0.5 0.50416667 0.50833333 0.5125 0.51666667 0.52083333 0.525 0.52916667 0.53333333 0.5375 0.54166667 0.54583333 0.55 0.55416667 0.55833333 0.5625 0.56666667 0.57083333 0.575 0.57916667 0.58333333 0.5875 0.59166667 0.59583333 0.6 0.60416667 0.60833333 0.6125 0.61666667 0.62083333 0.625 0.62916667 0.63333333 0.6375 0.64166667 0.64583333 0.65 0.65416667 0.65833333 0.6625 0.66666667 0.67083333 0.675 0.67916667 0.68333333 0.6875 0.69166667 0.69583333 0.7 0.70416667 0.70833333 0.7125 0.71666667 0.72083333 0.725 0.72916667 0.73333333 0.7375 0.74166667 0.74583333 0.75 0.75416667 0.75833333 0.7625 0.76666667 0.77083333 0.775 0.77916667 0.78333333 0.7875 0.79166667 0.79583333 0.8 0.80416667 0.80833333 0.8125 0.81666667 0.82083333 0.825 0.82916667 0.83333333 0.8375 0.84166667 0.84583333 0.85 0.85416667 0.85833333 0.8625 0.86666667 0.87083333 0.875 0.87916667 0.88333333 0.8875 0.89166667 0.89583333 0.9 0.90416667 0.90833333 0.9125 0.91666667 0.92083333 0.925 0.92916667 0.93333333 0.9375 0.94166667 0.94583333 0.95 0.95416667 0.95833333 0.9625 0.96666667 0.97083333 0.975 0.97916667 0.98333333 0.9875 0.99166667 0.99583333 1 1 1 1 1 1
  arc A47 (-7.4607, 2.2754) -> (-7.5989, 1.7598) centre (0, 0) ccw